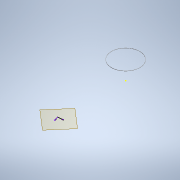
# Autodesk Inventor part: 零件3
Saved by Autodesk Inventor 2020 (Build 240168000, 168)
## iProperties
Created: 2021-06-27
Part Number: 零件3
Material: 常规
Document SubType Name: Modeling
Designer: chenpeizhi66
Density: 1 g/cm^3
Appearance: 默认
Author: chenpeizhi66
Autodesk Inventor part; units mm, degrees
ref_plane "YZ Plane" through (0, 0, 0) normal (1, 0, 0) x (0, 1, 0)
ref_plane "XZ Plane" through (0, 0, 0) normal (0, 1, 0) x (-1, 0, 0)
sketch "草图1" plane through (0, 0, 0) normal (0, 0, 1) x (1, 0, 0)
  circle A0 centre (0, 0) radius 75 projected
  circle A1 centre (0, 0) radius 74 projected
  point P0 (0, 0)
ref_plane "工作平面1" through (-136.6024, -136.6024, -1.225) normal (0, 0, 1) x (0.866, -0.5, 0)
extrude "拉伸1" add sketch "草图1" against normal up to surface (1.225 mm away)
ref_plane "工作平面2" through (0, -354, -97.405) normal (0, 0, 1) x (0.7578, -0.6525, 0)
sketch "草图2" plane through (0, -354, -97.405) normal (0, 0, 1) x (0.7578, -0.6525, 0)
  line L0 (2.923, 16.6348) -> (0.3965, 14.0501)
  line L1 (4.0671, 15.5163) -> (0.8949, 12.2711)
  line L2 (-0.8949, 12.7289) -> (-4.0671, 9.4837)
  line L3 (-0.3965, 10.9499) -> (-2.923, 8.3652)
  line L4 (-4.0172, -9.4175) -> (-0.8381, -11.1371)
  line L5 (-4.7785, -10.8248) -> (-0.7869, -12.9839)
  line L6 (0.7869, -12.0161) -> (4.7785, -14.1752)
  line L7 (0.8381, -13.8629) -> (4.0172, -15.5825)
  line L8 (5.3856, 18.0096) -> (-15.9852, -3.8534)
  line L9 (6.7939, -16.1749) -> (-15.9852, -3.8534)
  line L10 (4.0172, -13.7634) -> (3.256, -15.1708)
  line L11 (3.6366, 15.0759) -> (2.4924, 16.1943)
  point P0 (-230.9741, 268.2666)
  point P1 (3.6366, -14.4671)
  point P2 (3.0645, 15.6351)
  constraints: 24 end point, 6 point on line, 2 midpoint, 2 perpendicular, 1 parallel, 24 other
ref_plane "工作平面3" through (12.8896, -341.222, -99.2549) normal (0.9963, 0.0858, 0) x (0, 0, 1)
sketch "草图4" plane through (12.8896, -341.222, -99.2549) normal (0.9963, 0.0858, 0) x (0, 0, 1)
  circle A0 centre (1.9999, 2.8868) radius 0.8 projected
  circle A1 centre (1.9999, 2.8868) radius 0.8
  point P0 (99.2549, -341.069)
  constraints: 1 centre point, 1 coincident, 1 concentric
sweep "扫掠1" add profiles "草图4" path "草图2" path curves L8 L9
